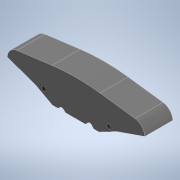
# Autodesk Inventor part: bumper
Saved by Autodesk Inventor 2022.2 (Build 262287000, 287)
## iProperties
Created: 2022-02-22
Part Number: bumper
Material: Polystyrene, Expanded
Document SubType Name: Modeling
Designer: hugof
Density: 0.05 g/cm^3
Appearance: Gray
Author: hugof
Autodesk Inventor part; units mm, degrees
ref_plane "YZ Plane" through (0, 0, 0) normal (1, 0, 0) x (0, 1, 0)
ref_plane "XZ Plane" through (0, 0, 0) normal (0, 1, 0) x (-1, 0, 0)
ref_plane "XY Plane" through (0, 0, 0) normal (0, 0, 1) x (1, 0, 0)
sketch "Sketch1" plane through (0, 0, 0) normal (0, 0, 1) x (1, 0, 0)
  line L0 (0, 0) -> (-4.8968, 0)
  line L1 (-14.75, 0) -> (-14.75, 2.0438)
  line L2 (-14.75, 4) -> (-7.375, 4)
  line L3 (0, 4) -> (0, 3.0438)
  line L4 (-10.875, 1) -> (-3.875, 1)
  line L5 (-10.875, 1) -> (-11.75, 1)
  line L6 (-3.875, 1) -> (-3, 1)
  line L7 (-9.8968, 0) -> (-9.2403, 0)
  line L8 (-14.75, 0) -> (-9.8968, 0)
  line L9 (-4.8968, 0) -> (0, 0)
  line L10 (-14.75, 1) -> (-11.75, 1)
  line L11 (0, 1) -> (-3, 1)
  line L12 (-9.8968, 0) -> (-11.75, 1)
  line L13 (-4.8968, 0) -> (-3, 1)
  line L14 (-11.75, 1) -> (-14.75, 1)
  line L15 (-3, 1) -> (0, 1)
  circle A0 centre (-10.875, 1) radius 0.25
  circle A1 centre (-3.875, 1) radius 0.25
  line L16 (-14.75, 1) -> (-14.75, 2.0438)
  line L17 (-11.75, 1) -> (-14.75, 2.0438)
  line L18 (0, 1) -> (0, 2.0438)
  line L19 (0, 2.0438) -> (-14.75, 2.0438)
  line L20 (-3, 1) -> (0, 2.0438)
  line L21 (-14.75, 2.0438) -> (-14.75, 3.0438)
  line L22 (-14.75, 3.0438) -> (-7.375, 4)
  line L23 (0, 2.0438) -> (0, 3.0438)
  line L24 (-7.375, 4) -> (0, 3.0438)
  line L25 (0, 2.0438) -> (0, 0)
  line L26 (0, 3.0438) -> (0, 2.0438)
  line L27 (-14.75, 3.0438) -> (-14.75, 4)
  line L28 (-14.75, 2.0438) -> (-14.75, 3.0438)
  line L29 (-7.375, 4) -> (0, 4)
  line L30 (-8.8787, 0) -> (-5.8787, 0)
  line L31 (-8.8757, 0) -> (-5.8787, 0)
  line L32 (-8.8757, 0) -> (-8.8757, 0.6246)
  line L33 (-5.8787, 0) -> (-5.8787, 0.7006)
  line L34 (-5.8787, 0.7006) -> (-6.2877, 0)
  line L35 (-5.8787, 0.7006) -> (-5.5532, 0)
  line L36 (-8.8757, 0.6246) -> (-8.5856, 0)
  line L37 (-8.8757, 0.6246) -> (-9.2403, 0)
  line L38 (-5.8787, 0) -> (-4.8968, 0)
  line L39 (-9.2403, 0) -> (-14.75, 0)
  line L40 (-4.8968, 0) -> (-5.5532, 0)
  line L41 (-5.5532, 0) -> (-9.2403, 0)
  line L42 (-9.2403, 0) -> (-8.8757, 0)
  point P0 (-7.375, 0)
  dimension "d0" = 14.75
  dimension "d1" = 4
  dimension "d2" = 7
  dimension "d3" = 1
  dimension "d4" = 5
  dimension "d5" = 3
  dimension "d6" = 3
  dimension "d7" = 0.5
  dimension "d8" = 0.5
  dimension "d9" = 1
  dimension "d10" = 3
  constraints: 86 end point, 19 parallel, 19 perpendicular, 13 point on line, 8 horizontal, 4 collinear, 3 equal length, 2 centre point, 2 coincident, 2 vertical
  measures "d0" distance of L2.start L3.start
  measures "d1" distance of L1.start L2.start
  measures "d2" distance of L4.start L4.end
  measures "d3" distance from line of L4 point (-7.375, 0)
  measures "d4" distance of L0.end L7.start
  measures "d5" distance of L10.start L5.end
  measures "d6" distance of L11.start L6.end
  measures "d7" diameter of A0
  measures "d8" diameter of A1
  measures "d9" distance of L18.end L3.end
  measures "d10" distance of L30.start L30.end
extrude "Extrusion1" add sketch "Sketch1" along normal blind 3 contours L38 L35 L34 L30 L36 L37 L7 L12 L5 A0 L4 A1 L6 L13 | L6 A1 L4 A0 L5 L17 L19 L20 | L19 L21 L22 L24 L23
fillet "Fillet1" radius 20 1 edges at (-7.375, 4, 1.5)
fillet "Fillet2" radius 1.2 2 edges at (-14.75, 3.0438, 1.5) (0, 3.0438, 1.5)
fillet "Fillet3" radius 2 2 edges at (-11.75, 1, 1.5) (-3, 1, 1.5)
fillet "Fillet4" radius 0.3 8 edges at (-8.8757, 0.6246, 1.5) (-5.8787, 0.7006, 1.5) (-9.2403, 0, 1.5) (-8.5856, 0, 1.5) (-6.2877, 0, 1.5) (-5.5532, 0, 1.5) (-4.8968, 0, 1.5) (-9.8968, 0, 1.5)
body "Solid1"
